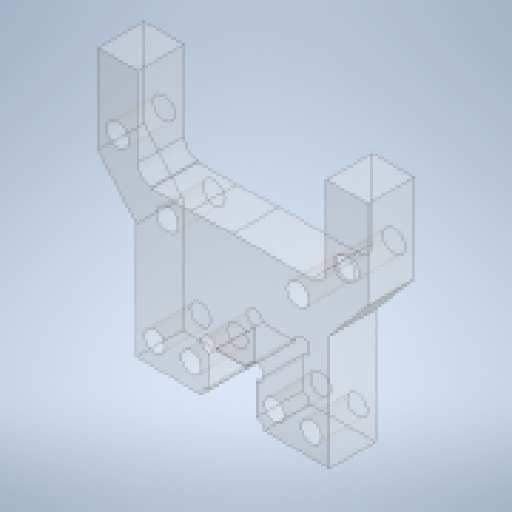
# Autodesk Inventor part: arm_connect_5
Saved by Autodesk Inventor 2024 (Build 280153000, 153)
## iProperties
Created: 2024-09-06
Part Number: arm_connect_5
Material: PMMA 플라스틱
Document SubType Name: Modeling
Designer: Eungang
Density: 1.188 g/cm^3
Appearance: 폴리카보네이트 - 선명
Mass: 4.05923 g
Surface Area: 25.7172 cm^2
Volume: 3.41686 cm^3
Author: Eungang
Autodesk Inventor part; units mm, degrees
ref_plane "YZ Plane" through (0, 0, 0) normal (1, 0, 0) x (0, 1, 0)
ref_plane "XZ Plane" through (0, 0, 0) normal (0, 1, 0) x (-1, 0, 0)
ref_plane "XY Plane" through (0, 0, 0) normal (0, 0, 1) x (1, 0, 0)
sketch "스케치1" plane through (0, 0, 0) normal (0, 0, 1) x (1, 0, 0)
  line L0 (7.15, 10.1828) -> (7.15, 9)
  arc A0 (7.15, 9) -> (9.15, 7) centre (9.15, 9) ccw
  line L1 (9.15, 7) -> (11.2, 7)
  arc A1 (12.2, 6) -> (11.2, 7) centre (11.2, 6) ccw
  line L2 (12.2, 6) -> (12.2, -27)
  line L3 (-12.2, -27) -> (-12.2, 6)
  arc A2 (-11.2, 7) -> (-12.2, 6) centre (-11.2, 6) ccw
  line L4 (-11.2, 7) -> (-9.15, 7)
  arc A3 (-9.15, 7) -> (-7.15, 9) centre (-9.15, 9) ccw
  line L5 (-7.15, 9) -> (-7.15, 10.1828)
  spline S0 degree 3 poles (-7.15, 10.1828) (-7.15, 10.4656) (-7.1021, 10.8015) (-6.9309, 11.2744) (-6.801, 11.5043) (-6.5407, 11.7954) (-6.3826, 11.9196) (-6.2267, 12) knots 0 0 0 0 0.420045 0.420045 0.746892 0.746892 1 1 1 1
  line L6 (-12.7, 12) -> (-6.2267, 12)
  line L7 (-17.8, 6) -> (-12.7, 12)
  line L8 (-17.8, -32.6) -> (-17.8, 6)
  line L9 (17.8, 6) -> (17.8, -32.6)
  line L10 (12.7, 12) -> (17.8, 6)
  line L11 (6.2267, 12) -> (12.7, 12)
  spline S1 degree 3 poles (6.2267, 12) (6.3826, 11.9196) (6.5407, 11.7954) (6.801, 11.5043) (6.9309, 11.2744) (7.1021, 10.8015) (7.15, 10.4656) (7.15, 10.1828) knots 0 0 0 0 0.253108 0.253108 0.579955 0.579955 1 1 1 1
  circle A4 centre (15, 4.5) radius 1.35
  circle A5 centre (-15, 4.5) radius 1.35
  line L12 (-10.5, -74.2) -> (10.5, -74.2)
  line L13 (10.5, -73.725) -> (10.5, -68.6)
  line L14 (10.5, -68.6) -> (13, -68.6)
  line L15 (13, -68.6) -> (15, -68.6)
  line L16 (15, -74.6) -> (15, -68.6)
  line L17 (10.5, -74.6) -> (10.5, -73.725)
  line L18 (-10.5, -73.725) -> (-10.5, -68.6)
  line L19 (-10.5, -74.6) -> (-10.5, -73.725)
  line L20 (-10.5, -68.6) -> (-13, -68.6)
  line L21 (-13, -68.6) -> (-15, -68.6)
  line L22 (-15, -74.6) -> (-15, -68.6)
  line L23 (-16.75, -74.2) -> (-15, -74.2)
  line L24 (-12.6075, -38.4) -> (-12.6075, -53.4)
  line L25 (-12.6075, -53.4) -> (12.6075, -53.4)
  line L26 (12.6075, -53.4) -> (12.6075, -38.4)
  line L27 (-3.0413, -53.4) -> (2.9587, -53.4)
  line L28 (-3.0413, -53.4) -> (2.9587, -53.4)
  line L29 (-3.1413, -53.5) -> (3.0587, -53.5)
  line L30 (3.0587, -53.5) -> (3.0587, -47.3)
  line L31 (3.0587, -47.3) -> (-3.1413, -47.3)
  line L32 (-3.1413, -47.3) -> (-3.1413, -53.5)
  circle A6 centre (-3.1413, -47.3) radius 1
  circle A7 centre (-3.1413, -53.4) radius 1
  circle A8 centre (3.0587, -47.3) radius 1
  circle A9 centre (3.0587, -53.4) radius 1
  circle A10 centre (7.8038, -50.4) radius 1.25
  circle A11 centre (-7.8037, -50.4) radius 1.25
  line L33 (21, -65.4) -> (-21, -65.4)
  line L34 (-21, -65.4) -> (-21, -59.4)
  line L35 (-12.6075, -59.4) -> (-21, -59.4)
  line L36 (-12.6075, -59.4) -> (-12.6075, -47.4)
  line L37 (12.6075, -47.4) -> (-12.6075, -47.4)
  line L38 (12.6075, -59.4) -> (12.6075, -47.4)
  line L39 (21, -59.4) -> (12.6075, -59.4)
  line L40 (21, -65.4) -> (21, -59.4)
  line L41 (12.7, 12) -> (9.2, 12)
  line L42 (12.7, 12) -> (17.8, 6)
  line L43 (17.8, 6) -> (17.8, -32.6)
  line L44 (17.8, -32.6) -> (12.7, -38.6)
  line L45 (12.7, -38.6) -> (-12.7, -38.6)
  line L46 (-12.7, -38.6) -> (-17.8, -32.6)
  line L47 (-17.8, -32.6) -> (-17.8, 6)
  line L48 (-17.8, 6) -> (-12.7, 12)
  line L49 (-9.2, 12) -> (-12.7, 12)
  arc A12 (-9.2, 12) -> (-12.2, 9) centre (-9.2, 9) ccw
  line L50 (-12.2, -30) -> (-12.2, 9)
  arc A13 (-12.2, -30) -> (-9.2, -33) centre (-9.2, -30) ccw
  line L51 (9.2, -33) -> (-9.2, -33)
  arc A14 (9.2, -33) -> (12.2, -30) centre (9.2, -30) ccw
  line L52 (12.2, 9) -> (12.2, -30)
  arc A15 (12.2, 9) -> (9.2, 12) centre (9.2, 9) ccw
  circle A16 centre (15, 4.5) radius 1.35
  circle A17 centre (15, -12.5) radius 1.35
  circle A18 centre (8.5, -35.8) radius 1.35
  circle A19 centre (-15, 4.5) radius 1.35
  circle A20 centre (-15, -12.5) radius 1.35
  circle A21 centre (-8.5, -35.8) radius 1.35
  circle A22 centre (15, -29.5) radius 1.35
  circle A23 centre (-15, -29.5) radius 1.35
  line L53 (-12.7, 11.8) -> (-10.7492, 11.8)
  arc A24 (-10.7492, 11.8) -> (-12.4, 9) centre (-9.2, 9) ccw
  line L54 (-12.4, 9) -> (-12.4, -30)
  arc A25 (-12.4, -30) -> (-9.2, -33.2) centre (-9.2, -30) ccw
  line L55 (-9.2, -33.2) -> (9.2, -33.2)
  arc A26 (9.2, -33.2) -> (12.4, -30) centre (9.2, -30) ccw
  line L56 (12.4, -30) -> (12.4, 9)
  arc A27 (12.4, 9) -> (10.7492, 11.8) centre (9.2, 9) ccw
  line L57 (10.7492, 11.8) -> (12.7, 11.8)
  line L58 (-17.6, -21) -> (-12.3919, -21)
  line L59 (-17.6, -21) -> (-17.8, -21)
  line L60 (17.5991, -21) -> (17.8, -21)
  line L61 (-12.3919, -21) -> (-12.2, -21)
  line L62 (12.4, -21) -> (12.2, -21)
  line L63 (12.4, -21) -> (17.5991, -21)
  point P0 (3.0587, -52.4)
  point P1 (4.0587, -53.4)
  point P2 (-4.1413, -53.4)
  point P3 (-3.1413, -52.4)
  point P4 (-3.1413, -48.3)
  point P5 (-2.1413, -47.3)
  point P6 (2.0587, -47.3)
  point P7 (3.0587, -48.3)
  point P8 (2.0637, -53.5)
  point P9 (2.0587, -53.4)
  point P10 (-2.1413, -53.4)
  point P11 (-2.1463, -53.5)
  point P12 (-2.1463, -47.4)
  point P13 (2.0637, -47.4)
  point P14 (12.6075, -38.6)
  point P15 (-12.4, -21)
  point P16 (-12.6075, -38.6)
  dimension "d6" = 15
  dimension "d8" = 2
  dimension "d9" = 2
  dimension "d10" = 2
  dimension "d11" = 2
  dimension "d43" = 0.2
  constraints: 36 end point, 13 point on line, 8 centre point, 8 point on circle, 4 perpendicular, 3 parallel, 2 coincident, 1 horizontal, 8 other
  measures "d6" distance of L24.end L24.start
  measures "d8" diameter of A6
  measures "d9" diameter of A7
  measures "d10" diameter of A8
  measures "d11" diameter of A9
  measures "d43" distance between parallel lines of L50 L54
extrude "돌출1" add sketch "스케치1" along normal blind 6 contours L9 L44 L45 L46 L8 L59 L58 L54 A25 L55 A26 L56 L63 L60 | L26 L37 A8 L31 A6 L24 L45 | L26 L25 A9 L30 A8 L37 | L37 A6 L32 A7 L25 L24 | L37 A6 L31 A8 | A10 | A11
sketch "스케치3" plane through (0, 0, 0) normal (0, 0, -1) x (-1, 0, 0)
  line L0 (3.1413, -52.4) -> (3.1413, -48.3) projected
  line L1 (12.6075, -38.6) -> (12.6075, -53.4) projected
  line L2 (7.8037, -50.4) -> (7.8037, -53.4)
  line L3 (12.6075, -53.4) -> (4.1413, -53.4) projected
  line L4 (7.8037, -50.4) -> (7.8037, -45.7034)
  line L5 (12.6075, -47.4) -> (-12.6075, -47.4) projected
  line L6 (-12.6075, -47.4) -> (-12.6075, -59.4) projected
  line L7 (-12.6075, -59.4) -> (12.6075, -59.4) projected
  line L8 (12.6075, -59.4) -> (12.6075, -47.4) projected
  line L9 (-12.6075, -53.4) -> (12.6075, -53.4)
  line L10 (4.1413, -53.4) -> (-12.6075, -53.4) projected
  line L11 (0, -53.4) -> (0, -47.4)
  circle A0 centre (10.2056, -50.4) radius 1.35
  circle A1 centre (5.4019, -50.4) radius 1.35
  circle A2 centre (-10.2056, -50.4) radius 1.35
  circle A3 centre (-5.4019, -50.4) radius 1.35
  point P0 (0, 0)
  point P1 (12.6075, -38.4)
  point P2 (-4.0587, -53.4)
  point P3 (-3.0587, -53.4)
  constraints: 8 end point, 4 centre point, 3 midpoint, 3 symmetric about line, 2 point on line, 1 collinear, 1 vertical, 2 other
extrude "돌출2" cut sketch "스케치3" against normal up to next contours A0 | A1 | A2 | A3
sketch "스케치4" plane through (0, 0, 0) normal (0, 0, -1) x (-1, 0, 0)
  circle A0 centre (-5.4019, -50.4) radius 1.35 projected
  circle A1 centre (5.4019, -50.4) radius 1.35 projected
  circle A2 centre (-10.2056, -50.4) radius 1.35 projected
  circle A3 centre (10.2056, -50.4) radius 1.35 projected
  line L0 (-3.0587, -48.3) -> (-3.0587, -52.4) projected
  arc A4 (-2.0637, -47.4) -> (-3.0587, -48.3) centre (-3.0587, -47.3) ccw projected
  arc A5 (3.1413, -48.3) -> (2.1463, -47.4) centre (3.1413, -47.3) ccw projected
  line L1 (3.1413, -52.4) -> (3.1413, -48.3) projected
  arc A6 (4.1413, -53.4) -> (3.1413, -52.4) centre (3.1413, -53.4) ccw projected
  line L2 (12.6075, -53.4) -> (4.1413, -53.4) projected
  arc A7 (-3.0587, -52.4) -> (-4.0587, -53.4) centre (-3.0587, -53.4) ccw projected
  line L3 (5.5223, -33.2046) -> (0, -33.2046)
  line L4 (0, -33.2046) -> (0, -33.4086)
  line L5 (0, -33.4086) -> (5.5223, -33.4086)
  line L6 (5.5223, -33.4086) -> (5.5223, -33.2046)
  line L7 (2.1463, -47.4) -> (-2.0637, -47.4) projected
  line L8 (12.6075, -38.6) -> (12.6075, -53.4) projected
  line L9 (12.7, -38.6) -> (12.6075, -38.6) projected
  line L10 (17.8, -32.6) -> (12.7, -38.6) projected
  line L11 (17.8, -21) -> (17.8, -32.6) projected
  line L12 (12.4, -21) -> (17.8, -21) projected
  line L13 (12.4, -30) -> (12.4, -21) projected
  arc A8 (9.2, -33.2) -> (12.4, -30) centre (9.2, -30) ccw projected
  line L14 (-9.2, -33.2) -> (9.2, -33.2) projected
  arc A9 (-12.4, -30) -> (-9.2, -33.2) centre (-9.2, -30) ccw projected
  line L15 (-12.4, -21) -> (-12.4, -30) projected
  line L16 (-17.8, -21) -> (-12.4, -21) projected
  line L17 (-17.8, -32.6) -> (-17.8, -21) projected
  line L18 (-12.7, -38.6) -> (-17.8, -32.6) projected
  line L19 (-12.6075, -38.6) -> (-12.7, -38.6) projected
  line L20 (-12.6075, -53.4) -> (-12.6075, -38.6) projected
  line L21 (-4.0587, -53.4) -> (-12.6075, -53.4) projected
  point P0 (0, 0)
  constraints: 8 end point, 2 parallel, 1 horizontal, 1 perpendicular
extrude "돌출3" add sketch "스케치4" against normal blind 6 contours L6 L5 L4 L3
sketch "스케치5" plane through (0, 0, 0) normal (0, 0, -1) x (-1, 0, 0)
  arc A0 (10.5959, -33.2046) -> (12.3919, -31.4086) centre (10.5959, -31.4086) ccw projected
  arc A1 (-12.2, -31.1962) -> (-10.2, -33.1962) centre (-10.2, -31.1962) ccw projected
  line L0 (10.5959, -33.2046) -> (-10.2, -33.1962)
  line L1 (10.5959, -33.2046) -> (-10.2001, -33.2046)
  line L2 (-10.2001, -33.2046) -> (-10.2001, -33.4742)
  line L3 (-10.2001, -33.4742) -> (10.5959, -33.4742)
  line L4 (10.5959, -33.4742) -> (10.5959, -33.2046)
  point P0 (0, 0)
  constraints: 10 end point, 2 parallel, 1 horizontal, 1 perpendicular, 1 tangent
extrude "돌출4" add sketch "스케치5" against normal blind 6
sketch "스케치6" plane through (0, 0, 0) normal (0, 0, -1) x (-1, 0, 0)
  line L0 (-10.2, -33.1962) -> (0, -33.1962) projected
  line L1 (0.2183, -33.2046) -> (10.5959, -33.2046) projected
  line L2 (-10.2, -33.1962) -> (10.5959, -33.1962)
  line L3 (10.5959, -33.1962) -> (10.5959, -33.2046)
  line L4 (10.5959, -33.2046) -> (-10.2, -33.2046)
  line L5 (-10.2, -33.2046) -> (-10.2, -33.1962)
  point P0 (0, 0)
  point P1 (0, -33.1962)
  constraints: 8 end point, 2 parallel, 1 horizontal, 1 perpendicular
extrude "돌출5" add sketch "스케치6" against normal blind 6
